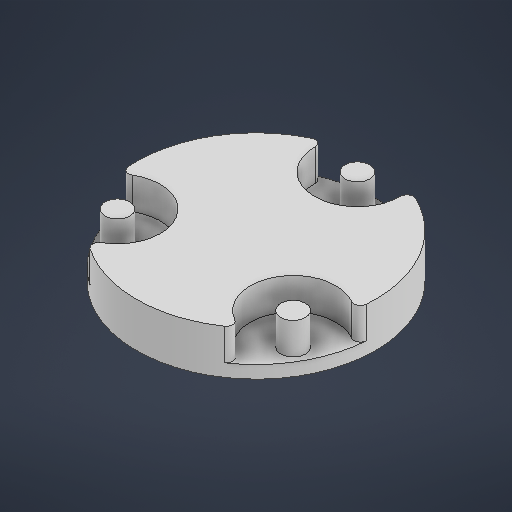
# Autodesk Inventor part: gewindeding
Saved by Autodesk Inventor 2026.2 (Build 302298000, 298)
## iProperties
Created: 2026-03-16
Part Number: gewindeding
Material: Generic
Document SubType Name: Modeling
Designer: Cobble
Density: 1 g/cm^3
Appearance: Default
Author: Cobble
Autodesk Inventor part; units mm, degrees
ref_plane "YZ Plane" through (0, 0, 0) normal (1, 0, 0) x (0, 1, 0)
ref_plane "XZ Plane" through (0, 0, 0) normal (0, 1, 0) x (-1, 0, 0)
ref_plane "XY Plane" through (0, 0, 0) normal (0, 0, 1) x (1, 0, 0)
sketch "Sketch1" plane through (0, 0, 0) normal (0, 0, 1) x (1, 0, 0)
  circle A0 centre (0, 0) radius 6.75
  circle A1 centre (0, 0) radius 1.95
  line L0 (0, 0) -> (0, -16)
  circle A2 centre (-13.8564, -24) radius 6.75
  circle A3 centre (-13.8564, -24) radius 1.95
  line L1 (-13.8564, -24) -> (0, -16)
  circle A4 centre (13.8564, -24) radius 6.75
  circle A5 centre (13.8564, -24) radius 1.95
  line L2 (13.8564, -24) -> (0, -16)
  circle A6 centre (0, -16) radius 18.85
  circle A7 centre (0, -16) radius 1.05
  circle A8 centre (0, -16) radius 4.75
  circle A9 centre (0, -20.75) radius 2.5
  circle A10 centre (4.1136, -13.625) radius 2.5
  circle A11 centre (-4.1136, -13.625) radius 2.5
  point P0 (18.5801, -19.1783)
  point P1 (6.5376, 1.68)
  point P2 (-6.5376, 1.68)
  point P3 (-18.5801, -19.1783)
  point P4 (-12.0425, -30.5017)
  point P5 (12.0425, -30.5017)
  dimension "d15" = 9.5
  dimension "d0" = 13.5
  dimension "d1" = 3.9
  dimension "d2" = 16
  dimension "d5" = 360
  dimension "d12" = 2.1
  dimension "d14" = 37.7
  dimension "d16" = 5
  dimension "d19" = 360
  constraints: 11 centre point, 10 coincident, 6 end point, 2 point on line, 1 vertical, 1 vertical alignment, 29 other
  measures "d0" diameter of A0
  measures "d1" diameter of A1
  measures "d2" distance of L0.start L0.end
  measures "d12" diameter of A7
  measures "d14" diameter of A6
  measures "d16" diameter of A9
extrude "Extrusion1" add sketch "Sketch1" along normal blind 5 contours A0 A6 A4 L2 A8 A10 L0 | L0 A8 A11 L1 A2 A6 A0 | A8 A10 L2 A7 L0 | L0 A7 L1 A8 A11 | A7 L2 L0 | L0 L1 A7 | A10 A8 | A8 A10 | A11 A8 | A8 A11 | L1 A8 A9 L2 A4 A6 A2 | L2 A7 L1 | A7 L2 A8 A9 L1 | A9 A8 | A8 A9 | A1 | A3 | A5
extrude "Extrusion2" add sketch "Sketch1" against normal blind 2 contours A0 A6 | A0 A6 A4 L2 A8 A10 L0 | L0 A8 A11 L1 A2 A6 A0 | A8 A10 L2 A7 L0 | L0 A7 L1 A8 A11 | A2 A6 | A6 A4 | A10 A8 | A8 A10 | A11 A8 | A8 A11 | L1 A8 A9 L2 A4 A6 A2 | A7 L2 A8 A9 L1 | A9 A8 | A8 A9 | A1 | A3 | A5 picked at (3.5494, 1.6258) picked at (-17.0838, -21.7871) picked at (17.0771, -21.7793)
fillet "Fillet1" radius 1 6 edges at (-12.0425, -30.5017, 2.5) (-18.5801, -19.1783, 2.5) (18.5801, -19.1783, 2.5) (12.0425, -30.5017, 2.5) (6.5376, 1.68, 2.5) (-6.5376, 1.68, 2.5)
body "Solid1"
